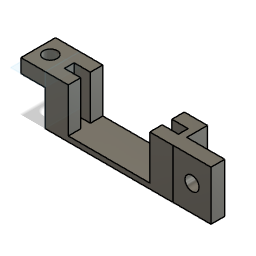
left motor v5 (Autodesk Fusion 360 design; units mm, degrees)
Autodesk Fusion 360 part; units mm, degrees
sketch "Esquisse1" plane through (0, 0, 0) normal (0, 1, 0) x (1, 0, 0)
  line L0 (0, 0) -> (36, 0)
  line L1 (36, 0) -> (36, -10)
  line L2 (36, -10) -> (0, -10)
  line L3 (0, -10) -> (0, 0)
  dimension "d1" = 36
  dimension "d2" = 10
  constraint horizontal L0
  constraint vertical L1
  constraint horizontal L2
  constraint vertical L3
  constraint coincident L0.start L3.end
  measures "d1" distance of L0.start L0.end
  measures "d2" distance of L0.start L2.end
sketch "Esquisse2" plane through (0, 1.5, 0) normal (0, 1, 0) x (-1, 0, 0)
  line L0 (0, 10) -> (-36, 10)
  line L1 (-36, 10) -> (-36, 0)
  line L2 (-36, 0) -> (0, 0)
  line L3 (0, 0) -> (0, 10)
  line L4 (0, 0) -> (-2, 0)
  line L5 (-2, 0) -> (-2, 10)
  line L6 (-2, 10) -> (0, 10)
  line L7 (0, 10) -> (0, 0)
  line L8 (-2, 0) -> (-6.7, 0)
  line L9 (-6.7, 0) -> (-6.7, 3.75)
  line L10 (-6.7, 3.75) -> (-2, 3.75)
  line L11 (-2, 3.75) -> (-2, 0)
  line L12 (-2, 10) -> (-6.7, 10)
  line L13 (-6.7, 10) -> (-6.7, 6.25)
  line L14 (-6.7, 6.25) -> (-2, 6.25)
  line L15 (-2, 6.25) -> (-2, 10)
  line L16 (-36, 0) -> (-34, 0)
  line L17 (-34, 0) -> (-34, 10)
  line L18 (-34, 10) -> (-36, 10)
  line L19 (-36, 10) -> (-36, 0)
  line L20 (-34, 0) -> (-29.3, 0)
  line L21 (-29.3, 0) -> (-29.3, 3.75)
  line L22 (-29.3, 3.75) -> (-34, 3.75)
  line L23 (-34, 3.75) -> (-34, 0)
  line L24 (-34, 10) -> (-29.3, 10)
  line L25 (-29.3, 10) -> (-29.3, 6.25)
  line L26 (-29.3, 6.25) -> (-34, 6.25)
  line L27 (-34, 6.25) -> (-34, 10)
  dimension "d5" = 2
  dimension "d6" = 4.7
  dimension "d7" = 3.75
  dimension "d8" = 4.7
  dimension "d9" = 3.75
  dimension "d10" = 2
  dimension "d11" = 4.7
  dimension "d12" = 3.75
  dimension "d13" = 4.7
  dimension "d14" = 3.75
  constraint horizontal L4
  constraint vertical L5
  constraint horizontal L6
  constraint vertical L7
  constraint coincident L2.end L3.start
  constraint horizontal L8
  constraint vertical L9
  constraint horizontal L10
  constraint vertical L11
  constraint horizontal L12
  constraint vertical L13
  constraint horizontal L14
  constraint vertical L15
  constraint horizontal L16
  constraint vertical L17
  constraint horizontal L18
  constraint vertical L19
  constraint coincident L1.end L2.start
  constraint horizontal L20
  constraint vertical L21
  constraint horizontal L22
  constraint vertical L23
  constraint horizontal L24
  constraint vertical L25
  constraint horizontal L26
  constraint vertical L27
  measures "d5" distance of L2.end L4.end
  measures "d6" distance of L4.end L8.end
  measures "d7" distance of L4.end L10.end
  measures "d8" distance of L5.end L12.end
  measures "d9" distance of L5.end L14.end
  measures "d10" distance of L1.end L16.end
  measures "d11" distance of L16.end L20.end
  measures "d12" distance of L16.end L22.end
  measures "d13" distance of L17.end L24.end
  measures "d14" distance of L17.end L26.end
sketch "Esquisse3" plane through (0, 0, 0) normal (0, 1, 0) x (1, 0, 0)
  line L0 (0, 0) -> (36.1, 0)
  line L1 (36.1, 0) -> (36.1, -10)
  line L2 (36.1, -10) -> (0, -10)
  line L3 (0, -10) -> (0, 0)
  dimension "d17" = 36.1
  dimension "d18" = 10
  constraint horizontal L0
  constraint vertical L1
  constraint horizontal L2
  constraint vertical L3
  constraint coincident L0.start L3.end
  measures "d17" distance of L0.start L0.end
  measures "d18" distance of L0.start L2.end
sketch "Esquisse4" plane through (0, 1.5, 0) normal (0, 1, 0) x (-1, 0, 0)
  line L0 (0, 10) -> (-36.1, 10)
  line L1 (-36.1, 10) -> (-36.1, 0)
  line L2 (-36.1, 0) -> (0, 0)
  line L3 (0, 0) -> (0, 10)
  line L4 (0, 0) -> (-2, 0)
  line L5 (-2, 0) -> (-2, 10)
  line L6 (-2, 10) -> (0, 10)
  line L7 (0, 10) -> (0, 0)
  line L8 (-36.1, 0) -> (-34.1, 0)
  line L9 (-34.1, 0) -> (-34.1, 10)
  line L10 (-34.1, 10) -> (-36.1, 10)
  line L11 (-36.1, 10) -> (-36.1, 0)
  line L12 (-2, 0) -> (-6.7, 0)
  line L13 (-6.7, 0) -> (-6.7, 3.75)
  line L14 (-6.7, 3.75) -> (-2, 3.75)
  line L15 (-2, 3.75) -> (-2, 0)
  line L16 (-2, 10) -> (-6.7, 10)
  line L17 (-6.7, 10) -> (-6.7, 6.25)
  line L18 (-6.7, 6.25) -> (-2, 6.25)
  line L19 (-2, 6.25) -> (-2, 10)
  line L20 (-34.1, 0) -> (-29.4, 0)
  line L21 (-29.4, 0) -> (-29.4, 3.75)
  line L22 (-29.4, 3.75) -> (-34.1, 3.75)
  line L23 (-34.1, 3.75) -> (-34.1, 0)
  line L24 (-34.1, 10) -> (-29.4, 10)
  line L25 (-29.4, 10) -> (-29.4, 6.25)
  line L26 (-29.4, 6.25) -> (-34.1, 6.25)
  line L27 (-34.1, 6.25) -> (-34.1, 10)
  dimension "d21" = 2
  dimension "d22" = 2
  dimension "d23" = 4.7
  dimension "d24" = 3.75
  dimension "d25" = 4.7
  dimension "d26" = 3.75
  dimension "d27" = 4.7
  dimension "d28" = 3.75
  dimension "d29" = 4.7
  dimension "d30" = 3.75
  constraint horizontal L4
  constraint vertical L5
  constraint horizontal L6
  constraint vertical L7
  constraint coincident L2.end L3.start
  constraint horizontal L8
  constraint vertical L9
  constraint horizontal L10
  constraint vertical L11
  constraint coincident L1.end L2.start
  constraint horizontal L12
  constraint vertical L13
  constraint horizontal L14
  constraint vertical L15
  constraint horizontal L16
  constraint vertical L17
  constraint horizontal L18
  constraint vertical L19
  constraint horizontal L20
  constraint vertical L21
  constraint horizontal L22
  constraint vertical L23
  constraint horizontal L24
  constraint vertical L25
  constraint horizontal L26
  constraint vertical L27
  measures "d21" distance of L2.end L4.end
  measures "d22" distance of L1.end L8.end
  measures "d23" distance of L4.end L12.end
  measures "d24" distance of L4.end L14.end
  measures "d25" distance of L5.end L16.end
  measures "d26" distance of L5.end L18.end
  measures "d27" distance of L8.end L20.end
  measures "d28" distance of L8.end L22.end
  measures "d29" distance of L9.end L24.end
  measures "d30" distance of L9.end L26.end
sketch "Esquisse5" plane through (0, 0, 0) normal (0, 1, 0) x (1, 0, 0)
  line L0 (0, 0) -> (37, 0)
  line L1 (37, 0) -> (37, -10)
  line L2 (37, -10) -> (0, -10)
  line L3 (0, -10) -> (0, 0)
  dimension "d33" = 37
  dimension "d34" = 10
  constraint horizontal L0
  constraint vertical L1
  constraint horizontal L2
  constraint vertical L3
  constraint coincident L0.start L3.end
  measures "d33" distance of L0.start L0.end
  measures "d34" distance of L0.start L2.end
extrude "Extrusion5" add sketch "Esquisse5" along normal blind 1.5
sketch "Esquisse6" plane through (0, 1.5, 0) normal (0, 1, 0) x (-1, 0, 0)
  line L0 (0, 10) -> (-37, 10)
  line L1 (-37, 10) -> (-37, 0)
  line L2 (-37, 0) -> (0, 0)
  line L3 (0, 0) -> (0, 10)
  line L4 (0, 0) -> (-2, 0)
  line L5 (-2, 0) -> (-2, 10)
  line L6 (-2, 10) -> (0, 10)
  line L7 (0, 10) -> (0, 0)
  line L8 (-37, 0) -> (-35, 0)
  line L9 (-35, 0) -> (-35, 10)
  line L10 (-35, 10) -> (-37, 10)
  line L11 (-37, 10) -> (-37, 0)
  line L12 (-2, 0) -> (-6.7, 0)
  line L13 (-6.7, 0) -> (-6.7, 3.6)
  line L14 (-6.7, 3.6) -> (-2, 3.6)
  line L15 (-2, 3.6) -> (-2, 0)
  line L16 (-2, 10) -> (-6.7, 10)
  line L17 (-6.7, 10) -> (-6.7, 6.4)
  line L18 (-6.7, 6.4) -> (-2, 6.4)
  line L19 (-2, 6.4) -> (-2, 10)
  line L20 (-35, 0) -> (-30.3, 0)
  line L21 (-30.3, 0) -> (-30.3, 3.6)
  line L22 (-30.3, 3.6) -> (-35, 3.6)
  line L23 (-35, 3.6) -> (-35, 0)
  line L24 (-35, 10) -> (-30.3, 10)
  line L25 (-30.3, 10) -> (-30.3, 6.4)
  line L26 (-30.3, 6.4) -> (-35, 6.4)
  line L27 (-35, 6.4) -> (-35, 10)
  dimension "d37" = 2
  dimension "d38" = 2
  dimension "d39" = 4.7
  dimension "d40" = 3.6
  dimension "d41" = 4.7
  dimension "d42" = 3.6
  dimension "d43" = 4.7
  dimension "d44" = 3.6
  dimension "d45" = 4.7
  dimension "d46" = 3.6
  constraint horizontal L4
  constraint vertical L5
  constraint horizontal L6
  constraint vertical L7
  constraint coincident L2.end L3.start
  constraint horizontal L8
  constraint vertical L9
  constraint horizontal L10
  constraint vertical L11
  constraint coincident L1.end L2.start
  constraint horizontal L12
  constraint vertical L13
  constraint horizontal L14
  constraint vertical L15
  constraint horizontal L16
  constraint vertical L17
  constraint horizontal L18
  constraint vertical L19
  constraint horizontal L20
  constraint vertical L21
  constraint horizontal L22
  constraint vertical L23
  constraint horizontal L24
  constraint vertical L25
  constraint horizontal L26
  constraint vertical L27
  measures "d37" distance of L2.end L4.end
  measures "d38" distance of L1.end L8.end
  measures "d39" distance of L4.end L12.end
  measures "d40" distance of L4.end L14.end
  measures "d41" distance of L5.end L16.end
  measures "d42" distance of L5.end L18.end
  measures "d43" distance of L8.end L20.end
  measures "d44" distance of L8.end L22.end
  measures "d45" distance of L9.end L24.end
  measures "d46" distance of L9.end L26.end
extrude "Extrusion6" add sketch "Esquisse6" along normal blind 12.5 contours L0 L2 L3 L4 L5 L6 L7 L15 L19 | L0 L5 L16 L17 L18 L19 | L2 L5 L12 L13 L14 L15 | L0 L9 L24 L25 L26 L27 | L0 L1 L2 L8 L9 L10 L11 L23 L27 | L2 L9 L20 L21 L22 L23
extrude "Extrusion7" add 2 faces at (2.9, 14, 8.8) (34.1, 14, 1.2) along direction (0, 1, 0) blind 0.5
extrude "Extrusion8" cut 2 faces at (2.9, 14.5, 8.8) (34.1, 14.5, 1.2) along direction (0, -1, 0) blind 0.2
sketch "Esquisse7" plane through (37, 0, 0) normal (1, 0, 0) x (0, 0, -1)
  line L0 (0, 14.3) -> (-10, 14.3)
  line L1 (-10, 14.3) -> (-10, 0)
  line L2 (-10, 0) -> (0, 0)
  line L3 (0, 0) -> (0, 14.3)
  line L4 (-6.9686, 14.3) -> (-3, 14.3)
  line L5 (-3, 14.3) -> (-3, 0)
  line L6 (-3, 0) -> (-6.9686, 0)
  line L7 (-6.9686, 0) -> (-6.9686, 14.3)
  constraint horizontal L4
  constraint vertical L5
  constraint horizontal L6
  constraint vertical L7
  constraint coincident L2 L5.end
  constraint coincident L0 L4.start
extrude "Extrusion9" add sketch "Esquisse7" along normal blind 11 contours L0 L2 L4 L5 L6 L7
sketch "Esquisse8" plane through (0, 0, 6.9686) normal (0, 0, 1) x (1, 0, 0)
  line L0 (37, 14.3) -> (37, 0)
  line L1 (37, 0) -> (48, 0)
  line L2 (48, 0) -> (48, 14.3)
  line L3 (48, 14.3) -> (37, 14.3)
  circle A0 centre (42.5, 7.5) radius 2.05
  dimension "d55" = 4.1
  measures "d55" diameter of A0
extrude "Extrusion10" cut sketch "Esquisse8" against normal blind 8.5 contours A0
sketch "Esquisse9" plane through (0, 0, 0) normal (-1, 0, 0) x (0, 0, 1)
  line L0 (10, 14.3) -> (0, 14.3)
  line L1 (0, 14.3) -> (0, 0)
  line L2 (0, 0) -> (10, 0)
  line L3 (10, 0) -> (10, 14.3)
sketch "Esquisse10" plane through (0, 0, 0) normal (-1, 0, 0) x (0, 0, 1)
  line L0 (0, 14.3) -> (10, 14.3)
  line L1 (10, 14.3) -> (10, 10.3)
  line L2 (10, 10.3) -> (0, 10.3)
  line L3 (0, 10.3) -> (0, 14.3)
  dimension "d58" = 4
  constraint horizontal L0
  constraint vertical L1
  constraint horizontal L2
  constraint vertical L3
  measures "d58" distance of L0.start L2.end
extrude "Extrusion11" add sketch "Esquisse10" along normal blind 10
sketch "Esquisse11" plane through (0, 0, 0) normal (-1, 0, 0) x (0, 0, 1)
sketch "Esquisse12" plane through (0, 10.3, 0) normal (0, -1, 0) x (1, 0, 0)
  line L0 (0, 0) -> (0, 10)
  line L1 (0, 10) -> (-10, 10)
  line L2 (-10, 10) -> (-10, 0)
  line L3 (-10, 0) -> (0, 0)
extrude "Extrusion12" cut 1 faces at (-10, 12.9667, 3.3333) along direction (1, 0, 0) blind 3
sketch "Esquisse13" plane through (0, 10.3, 0) normal (0, -1, 0) x (1, 0, 0)
  circle A0 centre (-3.5, 5) radius 2
  dimension "d63" = 4
  measures "d63" diameter of A0
extrude "Extrusion13" cut sketch "Esquisse13" against normal blind 10
extrude "Extrusion14" add 1 faces at (42.4489, 1.8186, 6.9686) along direction (0, 0, 1) blind 3
extrude "Extrusion15" cut 1 faces at (42.4489, 1.8186, 3) along direction (0, 0, 1) blind 3
